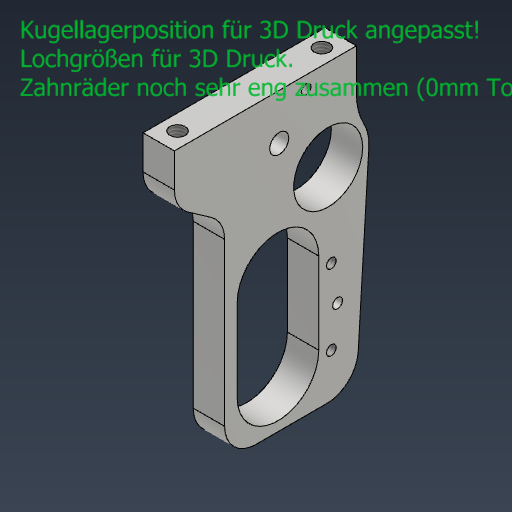
# Autodesk Inventor part: Dribbler Seite v2
Saved by Autodesk Inventor 2022.3 (Build 263350000, 350)
## iProperties
Part Number: Dribbler Seite v2
Material: Aluminium 6061
Document SubType Name: Modeling
Designer: rYan
Density: 2.7 g/cm^3
Appearance: Aluminium - flach
Mass: 9.16666 g
Surface Area: 28.695 cm^2
Volume: 3.39506 cm^3
Author: rYan
Autodesk Inventor part; units mm, degrees
ref_plane "YZ Plane" through (0, 0, 0) normal (1, 0, 0) x (0, 1, 0)
ref_plane "XZ Plane" through (0, 0, 0) normal (0, 1, 0) x (-1, 0, 0)
ref_plane "XY Plane" through (0, 0, 0) normal (0, 0, 1) x (1, 0, 0)
sketch "Skizze1" plane through (0, 0, 0) normal (1, 0, 0) x (0, 1, 0)
  circle A0 centre (-22.8, 48.7) radius 11 construction
  line L0 (-97.7565, 0) -> (58.6427, 0) projected
  circle A1 centre (14.8, 21.5) radius 21.5 construction
  line L1 (0, 10) -> (0, 33.674) construction
  line L2 (-6.7, 0) -> (-6.7, 21.5) construction
  circle A2 centre (-4.5, 42.5) radius 5 construction
  line L3 (-56.6136, 29) -> (0, 29) construction
  line L4 (-75.4137, 30) -> (0, 30) construction
  line L5 (-21, 43.3983) -> (-29, 49)
  line L6 (-29, 49) -> (-29, 57)
  circle A3 centre (-4.5, 42.5) radius 5.5
  circle A4 centre (-22.8, 48.7) radius 0.5
  circle A5 centre (-3, 23) radius 0.8
  line L7 (14.8, 21.5) -> (-6.7, 21.5) construction
  line L8 (-29, 57) -> (0, 57)
  line L9 (14.8, 21.5) -> (14.8, 20.5) construction
  line L10 (14.8, 20.5) -> (-4.5, 42.5) construction
  circle A6 centre (-22.8, 48.7) radius 4.95 construction
  circle A7 centre (-12.2958, 49.6823) radius 5.6 construction
  circle A8 centre (-12.2958, 49.6823) radius 6.3 construction
  circle A9 centre (-12.2958, 49.6823) radius 1.525
  line L11 (0, 50.374) -> (0, 57)
  line L12 (-21, 43.3983) -> (-21, 10)
  line L13 (-21, 10) -> (0, 10)
  arc A10 (1.9876, 42.0983) -> (1.2121, 45.6019) centre (-4.5, 42.5) ccw
  line L14 (1.9876, 42.0983) -> (0, 10)
  arc A11 (0, 50.374) -> (1.2121, 45.6019) centre (10, 50.374) ccw
  line L15 (-12.5, 18) -> (-12.5, 31) construction
  line L16 (-19, 18) -> (-19, 31)
  line L17 (-6, 31) -> (-6, 18)
  arc A12 (-19, 18) -> (-6, 18) centre (-12.5, 18) ccw
  arc A13 (-6, 31) -> (-19, 31) centre (-12.5, 31) ccw
  point P0 (0, 0)
  point P1 (-12.5, 24.5)
  dimension "d4" = 43
  dimension "d0" = 22
  dimension "d6" = 6.7
  dimension "d8" = 10
  dimension "d9" = 29
  dimension "d11" = 30
  dimension "d19" = 29
  dimension "d20" = 11
  dimension "d33" = 1
  dimension "d34" = 48.7
  dimension "d36" = 1.6
  dimension "d37" = 3
  dimension "d54" = 57
  dimension "d58" = 1
  dimension "d65" = 9.9
  dimension "d66" = 11.2
  dimension "d67" = 0.7
  dimension "d68" = 3.05
  dimension "d73" = 22.8
  dimension "d100" = 10.5042
  dimension "d101" = 0.9823
  dimension "d102" = 0
  dimension "d103" = 8.3
  dimension "d104" = 21
  dimension "d107" = 10
  dimension "d110" = 8
  dimension "d111" = 55
  dimension "d112" = 13
  dimension "d113" = 10
  dimension "d114" = 42.5
  dimension "d115" = 34
  dimension "d116" = 21
  dimension "d131" = 13
  dimension "d132" = 13
  dimension "d133" = 12.5
  dimension "d134" = 18
  dimension "d135" = 4.5
  dimension "d136" = 10.55
  constraints: 36 end point, 13 centre point, 9 tangent, 8 point on circle, 7 coincident, 4 horizontal, 4 point on line, 4 vertical, 3 perpendicular, 1 collinear, 1 horizontal alignment, 1 midpoint, 1 parallel, 2 other
  measures "d0" diameter of A0
  measures "d6" distance between parallel lines of L1 L2
  measures "d8" diameter of A2
  measures "d9" distance between parallel lines of L0 L3
  measures "d11" distance between parallel lines of L0 L4
  measures "d19" distance between parallel lines of L1 L6
  measures "d20" diameter of A3
  measures "d33" diameter of A4
  measures "d34" distance from line of L0 A0.centre
  measures "d36" diameter of A5
  measures "d37" distance from line of L1 A5.centre
  measures "d54" distance between parallel lines of L0 L8
  measures "d58" distance of L7.start L9.end
  measures "d65" diameter of A6
  measures "d66" diameter of A7
  measures "d67" radial gap between concentric circles of A8 A7
  measures "d68" diameter of A9
  measures "d73" distance from line of A0.centre L11
  measures "d100" horizontal distance of A7.centre A0.centre
  measures "d101" vertical distance of A7.centre A0.centre
  measures "d103" distance from line of A0.centre L8
  measures "d104" vertical distance of L7.start point (-4.5, 42.5)
  measures "d107" distance between parallel lines of L0 L13
  measures "d110" distance of L5.end L6.end
  measures "d111" angle of L5 L6
  measures "d112" diameter of A10
  measures "d113" radius of A11
  measures "d114" distance from line of L0 point (-4.5, 42.5)
  measures "d115" distance from line of A5.centre L8
  measures "d116" distance between parallel lines of L1 L12
  measures "d131" distance between parallel lines of L17 L16
  measures "d132" distance of L15.start L15.end
  measures "d133" distance between parallel lines of L1 L15
  measures "d134" distance from line of L0 L15.start
  measures "d135" distance from line of L1 L10.end
  measures "d136" distance of A8.centre A0.centre
extrude "Extrusion1" add sketch "Skizze1" along normal mid plane 5 contours L5 L6 L8 L11 A11 A10 L14 L13 L12 | A4
sketch "Skizze2" plane through (-2.5, -29, 57) normal (0, 0, 1) x (1, 0, 0)
  line L0 (0, 0) -> (5, 0) projected
  line L1 (5, 5) -> (5, 0) projected
  line L2 (0, 0) -> (0, 5) projected
  line L3 (2.5, 29) -> (2.5, 0) construction
  line L4 (0, 0) -> (5, 0) construction
  line L5 (0, 5) -> (5, 5) projected
  line L6 (0, 29) -> (5, 29) projected
  line L7 (0, 29) -> (5, 29) projected
  point P0 (2.5, 26)
  point P1 (2.5, 3)
  dimension "d25" = 23
  dimension "d74" = 3
  constraints: 2 end point, 2 point on line, 1 midpoint
  measures "d25" distance of point (2.5, 3) point (2.5, 26)
  measures "d74" distance from line of L6 point (2.5, 26)
hole "Bohrung1" at (0, -3, 57) at (0, -26, 57) direction (0, 0, -1) diameter 2.459 depth 7 tip angle 118 thread size "M3x0.5" class "6H" standard "ISO Metric profile"
sketch "Skizze3" plane through (-2.5, 0, 0) normal (-1, 0, 0) x (0, 0, 1)
  circle A0 centre (23, -3) radius 0.8 projected
  line L0 (29, -4) -> (17, -4) construction
  circle A1 centre (23, -3) radius 0.8 construction
  line L1 (23, -4) -> (23, -3) construction
  point P0 (0, 0)
  point P1 (55, -8)
  dimension "d38" = 12
  dimension "d39" = 1
  dimension "d40" = 32
  dimension "d41" = 5
  constraints: 4 end point, 2 coincident, 1 horizontal, 1 midpoint, 1 vertical
  measures "d38" distance of L0.start L0.end
  measures "d39" distance from line of L0 A0.centre
  measures "d40" horizontal distance of point (55, -8) A0.centre
  measures "d41" vertical distance of point (55, -8) A0.centre
hole "Bohrung2" at (-2.5, -4, 17) at (-2.5, -4, 29) at (-2.5, -8, 55) direction (1, 0, 0) diameter 1.567 end through all thread size "M2x0.4" class "6H" standard "ISO Metric profile"
fillet "Rundung3" radius 5 4 edges at (0, 0, 10) (0, -21, 10) (0, -21, 43.3983) (0, -29, 49)
